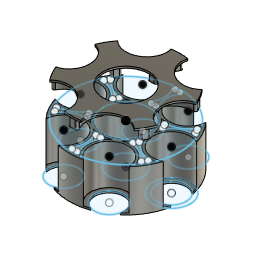
PingleCoinLoadForStore Roulette v2 (Autodesk Fusion 360 design; units mm, degrees)
Autodesk Fusion 360 part; units mm, degrees
note: some values were not read from the file. Chosen so that the rebuilt part matches the saved one: which bodies a step acts on. Set by a fixed rule: which sketch regions a step uses.
sketch "Sketch1" plane through (0, 0, 0) normal (0, 0, 1) x (1, 0, 0)
  circle A0 centre (0, 0) radius 31
  circle A1 centre (-25, 0) radius 10.25
  circle A2 centre (-12.5, -21.6506) radius 10.25
  circle A3 centre (12.5, -21.6506) radius 10.25
  circle A4 centre (25, 0) radius 10.25
  circle A5 centre (12.5, 21.6506) radius 10.25
  circle A6 centre (-12.5, 21.6506) radius 10.25
  dimension "d1" = 62
  dimension "d2" = 20.5
  dimension "d18" = 360
  constraint coincident A0.centre origin
  measures "d1" diameter of A0
  measures "d2" diameter of A1
extrude "Extrude1" add sketch "Sketch1" along normal blind 1.95 contours A0 A1 | A0 A1 makes body 1
pattern_linear "R-Pattern1" count 10 spacing 2.2222 along (0, 0, 1) of bodies 1 makes body 2 at (-22.7232, -1.8714, 2.2222) makes body 3 at (-22.7232, -1.8714, 4.4444) makes body 4 at (-22.7232, -1.8714, 6.6667) makes body 5 at (-22.7232, -1.8714, 8.8889) makes body 6 at (-22.7232, -1.8714, 11.1111) makes body 7 at (-22.7232, -1.8714, 13.3333) makes body 8 at (-22.7232, -1.8714, 15.5556) makes body 9 at (-22.7232, -1.8714, 17.7778) makes body 10 at (-22.7232, -1.8714, 20)
pattern_circular "C-Pattern1" count 6 over 360 about axis through (0, 0, 1.75) along (0, 0, 1) of bodies 7 9 8 10 5 1 6 3 4 2 makes body 11 at (-12.6618, -17.6369, 0) makes body 12 at (10.7134, -19.0584, 0) makes body 13 at (22.7232, 1.8714, 0) makes body 14 at (13.9763, 26.4195, 0) makes body 15 at (-8.3186, 25.3962, 0) makes body 16 at (-12.6618, -17.6369, 2.2222) makes body 17 at (10.7134, -19.0584, 2.2222) makes body 18 at (22.7232, 1.8714, 2.2222) makes body 19 at (13.9763, 26.4195, 2.2222) makes body 20 at (-8.3186, 25.3962, 2.2222) makes body 21 at (-12.6618, -17.6369, 4.4444) makes body 22 at (10.7134, -19.0584, 4.4444) makes body 23 at (22.7232, 1.8714, 4.4444) makes body 24 at (13.9763, 26.4195, 4.4444) makes body 25 at (-8.3186, 25.3962, 4.4444) makes body 26 at (-12.6618, -17.6369, 6.6667) makes body 27 at (10.7134, -19.0584, 6.6667) makes body 28 at (22.7232, 1.8714, 6.6667) makes body 29 at (13.9763, 26.4195, 6.6667) makes body 30 at (-8.3186, 25.3962, 6.6667) makes body 31 at (-12.6618, -17.6369, 8.8889) makes body 32 at (10.7134, -19.0584, 8.8889) makes body 33 at (22.7232, 1.8714, 8.8889) makes body 34 at (13.9763, 26.4195, 8.8889) makes body 35 at (-8.3186, 25.3962, 8.8889) makes body 36 at (-12.6618, -17.6369, 11.1111) makes body 37 at (10.7134, -19.0584, 11.1111) makes body 38 at (22.7232, 1.8714, 11.1111) makes body 39 at (13.9763, 26.4195, 11.1111) makes body 40 at (-8.3186, 25.3962, 11.1111) makes body 41 at (-12.6618, -17.6369, 13.3333) makes body 42 at (10.7134, -19.0584, 13.3333) makes body 43 at (22.7232, 1.8714, 13.3333) makes body 44 at (13.9763, 26.4195, 13.3333) makes body 45 at (-8.3186, 25.3962, 13.3333) makes body 46 at (-12.6618, -17.6369, 15.5556) makes body 47 at (10.7134, -19.0584, 15.5556) makes body 48 at (22.7232, 1.8714, 15.5556) makes body 49 at (13.9763, 26.4195, 15.5556) makes body 50 at (-8.3186, 25.3962, 15.5556) makes body 51 at (-12.6618, -17.6369, 17.7778) makes body 52 at (10.7134, -19.0584, 17.7778) makes body 53 at (22.7232, 1.8714, 17.7778) makes body 54 at (13.9763, 26.4195, 17.7778) makes body 55 at (-8.3186, 25.3962, 17.7778) makes body 56 at (-12.6618, -17.6369, 20) makes body 57 at (10.7134, -19.0584, 20) makes body 58 at (22.7232, 1.8714, 20) makes body 59 at (13.9763, 26.4195, 20) makes body 60 at (-8.3186, 25.3962, 20)
sketch "Sketch2" plane through (0, 0, 0) normal (0, 0, 1) x (1, 0, 0)
  arc A0 (22.7338, -21.0754) -> (6.8849, -30.2258) centre (12.5, -21.6506) ccw
  arc A1 (-6.8849, -30.2258) -> (6.8849, -30.2258) centre (0, 0) ccw
  arc A2 (-29.6187, -9.1504) -> (-22.7338, -21.0754) centre (0, 0) ccw
  arc A3 (-22.7338, 21.0754) -> (-29.6188, 9.1504) centre (0, 0) ccw
  arc A4 (6.8849, 30.2258) -> (-6.8849, 30.2258) centre (0, 0) ccw
  arc A5 (6.8849, 30.2258) -> (22.7338, 21.0754) centre (12.5, 21.6506) ccw
  arc A6 (22.7338, -21.0754) -> (29.6187, -9.1504) centre (0, 0) ccw
  arc A7 (29.6188, 9.1504) -> (22.7338, 21.0754) centre (0, 0) ccw
  arc A8 (29.6188, 9.1504) -> (29.6187, -9.1504) centre (25, 0) ccw
  arc A9 (-22.7338, 21.0754) -> (-6.8849, 30.2258) centre (-12.5, 21.6506) ccw
  arc A10 (-29.6187, -9.1504) -> (-29.6187, 9.1504) centre (-25, 0) ccw
  arc A11 (-6.8849, -30.2258) -> (-22.7338, -21.0754) centre (-12.5, -21.6506) ccw
  arc A12 (-3.9664, -29.434) -> (3.9664, -29.434) centre (0, 0) ccw
  arc A13 (23.5074, -18.152) -> (3.9664, -29.434) centre (12.5, -21.6506) ccw
  arc A14 (23.5074, -18.152) -> (27.4738, -11.282) centre (0, 0) ccw
  arc A15 (27.4738, 11.282) -> (27.4738, -11.282) centre (25, 0) ccw
  arc A16 (27.4738, 11.282) -> (23.5074, 18.152) centre (0, 0) ccw
  arc A17 (3.9664, 29.434) -> (23.5074, 18.152) centre (12.5, 21.6506) ccw
  arc A18 (3.9664, 29.434) -> (-3.9664, 29.434) centre (0, 0) ccw
  arc A19 (-23.5074, 18.152) -> (-3.9664, 29.434) centre (-12.5, 21.6506) ccw
  arc A20 (-23.5074, 18.152) -> (-27.4738, 11.282) centre (0, 0) ccw
  arc A21 (-27.4738, -11.282) -> (-27.4738, 11.282) centre (-25, 0) ccw
  arc A22 (-27.4738, -11.282) -> (-23.5074, -18.152) centre (0, 0) ccw
  arc A23 (-3.9664, -29.434) -> (-23.5074, -18.152) centre (-12.5, -21.6506) ccw
  dimension "d20" = 360
  dimension "d21" = 62
  dimension "d22" = 20.5
  dimension "d23" = 1.3
  constraint coincident A1.centre A2.centre
  constraint concentric A1 A6
  constraint concentric A2 A6
  constraint concentric A3 A6
  constraint concentric A4 A6
  constraint concentric A6 A7
  measures "d21" diameter of A6
  measures "d22" diameter of A10
sketch "Sketch3" plane through (0, 0, 0) normal (0, 0, 1) x (1, 0, 0)
  circle A0 centre (0, 0) radius 31
  constraint coincident A0.centre origin
extrude "Extrude4" add sketch "Sketch3" against normal blind 1 bodies 1 11 12 13 14 15
extrude "Extrude5" add sketch "Sketch2" along normal blind 25 separate body makes body 61
sketch "Sketch4" plane through (0, 0, 0) normal (0, 0, 1) x (1, 0, 0)
  circle A0 centre (0, 0) radius 12.5
  circle A1 centre (0, 0) radius 13.8
  dimension "d28" = 25
  dimension "d29" = 1.3
  constraint coincident A0.centre A1.centre
  measures "d28" diameter of A0
extrude "Extrude6" add sketch "Sketch4" along normal blind 25 bodies 61 1
extrude "Extrude7" cut 1 faces at (-6.2117, 12.1525, 25) along direction (0, 0, -1) blind 3.05 on bodies 61 bodies 61
sketch "Sketch5" plane through (0, 0, 0) normal (0, 0, 1) x (1, 0, 0)
sketch "Sketch6" plane through (0, 0, 0) normal (0, 0, 1) x (1, 0, 0)
extrude "Extrude8" cut 7 faces at (-13.5368, -8.2098, 0) (-0.3415, -15.8282, 0) (13.8783, -7.6183, 0) (-3.3879, -0.621, 0) (13.8783, 7.6183, 0) (0.3415, 15.8282, 0) (-13.5368, 8.2098, 0) along direction (0, 0, 1) blind -9 and the other way blind -32 on bodies 61 bodies 61
extrude "Extrude9" add sketch "Sketch4" against normal blind 1 contours A0 bodies 61
sketch "Sketch7" plane through (0, 0, 0) normal (0, 0, 1) x (1, 0, 0)
  circle A0 centre (25, 0) radius 10.25
  circle A1 centre (25, 0) radius 8
  circle A2 centre (12.5, 21.6506) radius 8
  circle A3 centre (-12.5, 21.6506) radius 8
  circle A4 centre (-25, 0) radius 8
  circle A5 centre (-12.5, -21.6506) radius 8
  circle A6 centre (12.5, -21.6506) radius 8
  circle A7 centre (0, 0) radius 9.2195
  dimension "d41" = 360
  dimension "d56" = 16
  constraint concentric A0 A1
  constraint coincident A7.centre origin
  measures "d56" diameter of A1
extrude "Extrude10" cut sketch "Sketch7" against normal blind 10 contours A1 | A2 | A3 | A4 | A5 | A6 bodies 61
extrude "Extrude11" cut 6 faces at (-8.5006, -22.188, 1.95) (10.2366, -23.8305, 1.95) (19.5069, -3.3941, 1.95) (15.5213, 23.5795, 1.95) (-13.0359, 26.6737, 1.95) (-25.2973, 3.2412, 1.95) along direction (0, 0, -1) blind 2 on bodies 61 bodies 61
extrude "Extrude12" cut sketch "Sketch7" against normal blind 6 contours A7 bodies 61
copy_body "CopyPasteBodies1" bodies 17 18 16 2 20 19 makes body 62 makes body 63 makes body 64 makes body 65 makes body 66 makes body 67
move_body "Move1" bodies 62 63 64 65 66 67 to x (1, 0, 0) y (0, 1, 0) z (0, 0, 1) at (0, 0, -2.1)
extrude "Extrude13" add sketch "Sketch1" along normal blind 21 separate body contours A0 A4 | A0 A4 | A0 A5 | A0 A5 | A0 A3 | A0 A3 | A0 A6 | A0 A6 | A0 A2 | A0 A2 | A0 A1 | A0 A1 makes body 68 at (35.1991, -1.0206, 7) makes body 69 at (-14.8009, -1.0206, 7) makes body 70 at (22.6991, -22.6712, 7) makes body 71 at (22.6991, 22.6712, 14) makes body 72 at (-2.3009, 20.6301, 7) makes body 73 at (-2.3009, -22.6712, 7)
extrude "Extrude14" cut 1 faces at (11.3257, -1.079, 0) along direction (0, 0, -1) blind 19 on bodies 61 bodies 61
sketch "Sketch8" plane through (0, 0, 0) normal (0, 0, 1) x (1, 0, 0)
  circle A0 centre (0, 0) radius 36
  dimension "d55" = 72
  constraint coincident A0.centre origin
  measures "d55" diameter of A0
sketch "Sketch9" plane through (0, 0, 0) normal (0, 0, 1) x (1, 0, 0)
sketch "Sketch10" plane through (0, 0, 0) normal (0, 0, 1) x (1, 0, 0)
sketch "Sketch11" plane through (0, 0, 21.95) normal (0, 0, 1) x (-1, 0, 0)
  arc A0 (-13.6407, 2.0904) -> (-27.4738, 11.282) centre (-25, 0) ccw
  arc A1 (-23.5074, 18.152) -> (-27.4738, 11.282) centre (0, 0) ccw
  arc A2 (-23.5074, 18.152) -> (-8.6307, 10.768) centre (-12.5, 21.6506) ccw
  arc A3 (-8.6307, 10.768) -> (-13.6407, 2.0904) centre (0, 0) ccw
  arc A4 (-13.6407, -2.0904) -> (-8.6307, -10.768) centre (0, 0) ccw
  arc A5 (-8.6307, -10.768) -> (-23.5074, -18.152) centre (-12.5, -21.6506) ccw
  arc A6 (-27.4738, -11.282) -> (-23.5074, -18.152) centre (0, 0) ccw
  arc A7 (-27.4738, -11.282) -> (-13.6407, -2.0904) centre (-25, 0) ccw
  arc A8 (-5.01, 12.8585) -> (-3.9664, 29.434) centre (-12.5, 21.6506) ccw
  arc A9 (3.9664, 29.434) -> (-3.9664, 29.434) centre (0, 0) ccw
  arc A10 (3.9664, 29.434) -> (5.01, 12.8585) centre (12.5, 21.6506) ccw
  arc A11 (5.01, 12.8585) -> (-5.01, 12.8585) centre (0, 0) ccw
  arc A12 (-5.01, -12.8585) -> (5.01, -12.8585) centre (0, 0) ccw
  arc A13 (5.01, -12.8585) -> (3.9664, -29.434) centre (12.5, -21.6506) ccw
  arc A14 (-3.9664, -29.434) -> (3.9664, -29.434) centre (0, 0) ccw
  arc A15 (-3.9664, -29.434) -> (-5.01, -12.8585) centre (-12.5, -21.6506) ccw
  arc A16 (8.6307, -10.768) -> (13.6408, -2.0904) centre (0, 0) ccw
  arc A17 (13.6408, -2.0904) -> (27.4737, -11.282) centre (25, 0) ccw
  arc A18 (23.5074, -18.152) -> (27.4738, -11.282) centre (0, 0) ccw
  arc A19 (23.5074, -18.152) -> (8.6307, -10.768) centre (12.5, -21.6506) ccw
  circle A20 centre (0, 0) radius 12.5
  arc A21 (-22.7338, 21.0754) -> (-29.6187, 9.1504) centre (0, 0) ccw
  arc A22 (-29.6188, -9.1504) -> (-29.6187, 9.1504) centre (-25, 0) ccw
  arc A23 (-29.6188, -9.1504) -> (-22.7338, -21.0754) centre (0, 0) ccw
  arc A24 (-6.8849, -30.2258) -> (-22.7338, -21.0754) centre (-12.5, -21.6506) ccw
  arc A25 (-6.8849, -30.2258) -> (6.8849, -30.2258) centre (0, 0) ccw
  arc A26 (22.7338, -21.0754) -> (6.8849, -30.2258) centre (12.5, -21.6506) ccw
  arc A27 (22.7338, -21.0754) -> (29.6188, -9.1504) centre (0, 0) ccw
  arc A28 (29.6188, 9.1504) -> (29.6187, -9.1504) centre (25, 0) ccw
  arc A29 (29.6188, 9.1504) -> (22.7338, 21.0754) centre (0, 0) ccw
  arc A30 (6.8849, 30.2258) -> (22.7338, 21.0754) centre (12.5, 21.6506) ccw
  arc A31 (6.8849, 30.2258) -> (-6.8849, 30.2258) centre (0, 0) ccw
  arc A32 (-22.7338, 21.0754) -> (-6.8849, 30.2258) centre (-12.5, 21.6506) ccw
  arc A33 (13.6408, 2.0904) -> (8.6307, 10.768) centre (0, 0) ccw
  arc A34 (8.6307, 10.768) -> (23.5074, 18.152) centre (12.5, 21.6506) ccw
  arc A35 (27.4738, 11.282) -> (23.5074, 18.152) centre (0, 0) ccw
  arc A36 (27.4737, 11.282) -> (13.6407, 2.0904) centre (25, 0) ccw
  arc A37 (-2.1679, 15.6465) -> (-2.2274, 27.756) centre (-12.5, 21.6506) ccw
  arc A38 (1.4161, 29.2658) -> (-1.4161, 29.2658) centre (0, 0) ccw
  arc A39 (2.2274, 27.756) -> (2.1679, 15.6465) centre (12.5, 21.6506) ccw
  arc A40 (1.2175, 14.1477) -> (-1.2175, 14.1477) centre (0, 0) ccw
  arc A41 (-1.4161, 29.2658) -> (-2.2274, 27.756) centre (-1.3677, 28.2669) ccw
  arc A42 (2.2274, 27.756) -> (1.4161, 29.2658) centre (1.3677, 28.2669) ccw
  arc A43 (1.2175, 14.1477) -> (2.1679, 15.6465) centre (1.3033, 15.144) ccw
  arc A44 (-2.1679, 15.6465) -> (-1.2175, 14.1477) centre (-1.3033, 15.144) ccw
  arc A45 (-11.6435, 8.1283) -> (-12.861, 6.0194) centre (0, 0) ccw
  arc A46 (-11.6435, 8.1283) -> (-12.4663, 9.7007) centre (-12.4635, 8.7007) ccw
  arc A47 (-22.9237, 15.807) -> (-12.4663, 9.7007) centre (-12.5, 21.6506) ccw
  arc A48 (-22.9237, 15.807) -> (-24.6369, 15.8592) centre (-23.796, 15.318) ccw
  arc A49 (-24.6369, 15.8592) -> (-26.0529, 13.4065) centre (0, 0) ccw
  arc A50 (-26.0529, 13.4065) -> (-25.1511, 11.949) centre (-25.1638, 12.949) ccw
  arc A51 (-14.6342, 5.9458) -> (-25.1511, 11.949) centre (-25, 0) ccw
  arc A52 (-14.6342, 5.9458) -> (-12.861, 6.0194) centre (-13.7667, 6.4433) ccw
  arc A53 (-12.861, -6.0194) -> (-11.6435, -8.1283) centre (0, 0) ccw
  arc A54 (-12.861, -6.0194) -> (-14.6342, -5.9458) centre (-13.7667, -6.4433) ccw
  arc A55 (-25.1511, -11.949) -> (-14.6342, -5.9458) centre (-25, 0) ccw
  arc A56 (-25.1511, -11.949) -> (-26.0529, -13.4065) centre (-25.1638, -12.949) ccw
  arc A57 (-26.0529, -13.4065) -> (-24.6369, -15.8592) centre (0, 0) ccw
  arc A58 (-24.6369, -15.8592) -> (-22.9237, -15.807) centre (-23.796, -15.318) ccw
  arc A59 (-12.4663, -9.7007) -> (-22.9237, -15.807) centre (-12.5, -21.6506) ccw
  arc A60 (-12.4663, -9.7007) -> (-11.6435, -8.1283) centre (-12.4635, -8.7007) ccw
  arc A61 (-1.2175, -14.1477) -> (1.2175, -14.1477) centre (0, 0) ccw
  arc A62 (-1.2175, -14.1477) -> (-2.1679, -15.6465) centre (-1.3033, -15.144) ccw
  arc A63 (-2.2274, -27.756) -> (-2.1679, -15.6465) centre (-12.5, -21.6506) ccw
  arc A64 (-2.2274, -27.756) -> (-1.4161, -29.2658) centre (-1.3677, -28.2669) ccw
  arc A65 (-1.4161, -29.2658) -> (1.4161, -29.2658) centre (0, 0) ccw
  arc A66 (1.4161, -29.2658) -> (2.2274, -27.756) centre (1.3677, -28.2669) ccw
  arc A67 (2.1679, -15.6465) -> (2.2274, -27.756) centre (12.5, -21.6506) ccw
  arc A68 (2.1679, -15.6465) -> (1.2175, -14.1477) centre (1.3033, -15.144) ccw
  arc A69 (11.6435, -8.1283) -> (12.861, -6.0194) centre (0, 0) ccw
  arc A70 (11.6435, -8.1283) -> (12.4663, -9.7007) centre (12.4635, -8.7007) ccw
  arc A71 (22.9237, -15.807) -> (12.4663, -9.7007) centre (12.5, -21.6506) ccw
  arc A72 (22.9237, -15.807) -> (24.6369, -15.8592) centre (23.796, -15.318) ccw
  arc A73 (24.6369, -15.8592) -> (26.0529, -13.4065) centre (0, 0) ccw
  arc A74 (26.0529, -13.4065) -> (25.1511, -11.949) centre (25.1637, -12.949) ccw
  arc A75 (14.6342, -5.9458) -> (25.1511, -11.949) centre (25, 0) ccw
  arc A76 (14.6342, -5.9458) -> (12.861, -6.0194) centre (13.7667, -6.4433) ccw
  arc A77 (12.861, 6.0194) -> (11.6435, 8.1283) centre (0, 0) ccw
  arc A78 (12.861, 6.0194) -> (14.6342, 5.9458) centre (13.7667, 6.4433) ccw
  arc A79 (25.1511, 11.949) -> (14.6342, 5.9458) centre (25, 0) ccw
  arc A80 (25.1511, 11.949) -> (26.0529, 13.4065) centre (25.1638, 12.949) ccw
  arc A81 (26.0529, 13.4065) -> (24.6369, 15.8592) centre (0, 0) ccw
  arc A82 (24.6369, 15.8592) -> (22.9237, 15.807) centre (23.796, 15.318) ccw
  arc A83 (12.4663, 9.7007) -> (22.9237, 15.807) centre (12.5, 21.6506) ccw
  arc A84 (12.4663, 9.7007) -> (11.6435, 8.1283) centre (12.4635, 8.7007) ccw
  circle A85 centre (0, 0) radius 29.7
  circle A86 centre (0, 0) radius 12.5
  dimension "d58" = 1
  dimension "d60" = 360
  constraint concentric A8 A37
  constraint concentric A9 A38
  constraint concentric A10 A39
  constraint concentric A11 A40
  constraint tangent A37 A41
  constraint tangent A38 A41
  constraint tangent A38 A42
  constraint tangent A39 A42
  constraint equal A41 A42
  constraint tangent A39 A43
  constraint tangent A40 A43
  constraint equal A41 A43
  constraint tangent A40 A44
  constraint tangent A37 A44
  constraint equal A41 A44
  constraint concentric A49 A85
  constraint concentric A45 A86
  measures "d58" radius of A41
extrude "Extrude15" add sketch "Sketch11" against normal blind 5 separate body contours A37 A38 A39 A40 A41 A42 A43 A44 | A45 A46 A47 A48 A49 A50 A51 A52 | A53 A54 A55 A56 A57 A58 A59 A60 | A61 A62 A63 A64 A65 A66 A67 A68 | A69 A70 A71 A72 A73 A74 A75 A76 | A77 A78 A79 A80 A81 A82 A83 A84 makes body 74 at (-12.9953, 9.7109, 18.6167) makes body 75 at (15.0911, -9.9849, 18.6167) makes body 76 at (-1.7277, 26.8236, 18.6167) makes body 77 at (-15.2006, -6.8392, 18.6167) makes body 78 at (-1.6774, -16.5838, 18.6167) makes body 79 at (21.4994, 11.4258, 18.6167)
extrude "Extrude16" add sketch "Sketch11" 6 faces at (-23.5868, 13.7996, 21.95) (0.1574, -27.3265, 21.95) (-0.1574, 27.3265, 21.95) (23.5868, 13.7996, 21.95) (-23.5868, -13.7996, 21.95) (23.7442, -13.527, 21.95) along normal blind 1 contours A0 A2 A3 A4 A5 A7 A8 A10 A11 A12 A13 A15 A16 A17 A19 A22 A24 A26 A28 A30 A32 A33 A34 A36 A85 | A0 A1 A2 A3 A85 | A22 A85 | A32 A85 | A4 A5 A6 A7 A85 | A8 A9 A10 A11 A85 | A24 A85 | A30 A85 | A12 A13 A14 A15 A85 | A33 A34 A35 A36 A85 | A26 A85 | A28 A85 | A16 A17 A18 A19 A85 | A37 A38 A39 A40 A41 A42 A43 A44 | A45 A46 A47 A48 A49 A50 A51 A52 | A53 A54 A55 A56 A57 A58 A59 A60 | A61 A62 A63 A64 A65 A66 A67 A68 | A69 A70 A71 A72 A73 A74 A75 A76 | A77 A78 A79 A80 A81 A82 A83 A84 on bodies 74 75 76 77 78 79 bodies 74 75 76 77 78 79
sketch "Sketch12" plane through (0, 0, 0) normal (0, 0, 1) x (1, 0, 0)
  ellipse E0 centre (30, 0) end of major axis (30, -11) minor radius 10.1695
  line L0 (30, 11) -> (30, -11)
  line L1 (19.8305, 0) -> (40.1695, 0)
  ellipse E1 centre (15, 25.9808) end of major axis (24.5263, 20.4808) minor radius 10.1695
  ellipse E2 centre (-15, 25.9808) end of major axis (-5.4737, 31.4808) minor radius 10.1695
  ellipse E3 centre (-30, 0) end of major axis (-30, 11) minor radius 10.1695
  ellipse E4 centre (-15, -25.9808) end of major axis (-24.5263, -20.4808) minor radius 10.1695
  ellipse E5 centre (15, -25.9808) end of major axis (5.4737, -31.4808) minor radius 10.1695
  dimension "d66" = 360
  constraint coincident E0 L0.start
  constraint coincident E0 L0.end
  constraint coincident E0 L1.start
  constraint coincident E0 L1.end
  constraint vertical L0
extrude "Extrude17" cut sketch "Sketch12" along normal blind 70 bodies 74
move_body "Move2" bodies 74 to x (1, 0, 0) y (0, 1, 0) z (0, 0, 1) at (0, 0, 16)
hidden bodies 68 69 70 71 72 73
equation "d61 = -2 mm - 3 mm"
named bodies: "Coin 10 cent EU holder"
